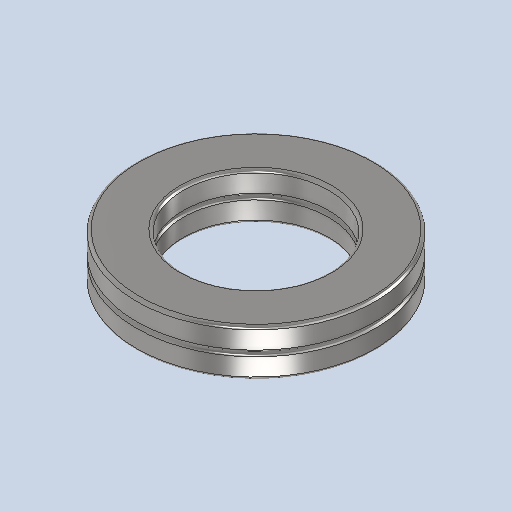
# Autodesk Inventor part: RB2508UUC0
Saved by Autodesk Inventor 2024.2 (Build 282272000, 272)
## iProperties
Created: 2024-01-04
Part Number: RB2508UUC0
Material: Generic
Document SubType Name: Modeling
Designer: Masato Kubotera
Density: 7.58662 g/cm^3
Appearance: Semi-Polished
Mass: 50 g
Surface Area: 33.4688 cm^2
Volume: 6.59055 cm^3
Catalog Web Link: https://jp.misumi-ec.com/vona2/detail/221000091353/?ProductCode=RB2508UUC0
Vendor: THK
Author: Masato Kubotera
Autodesk Inventor part; units mm, degrees
ref_plane "YZ Plane" through (0, 0, 0) normal (1, 0, 0) x (0, 1, 0)
ref_plane "XZ Plane" through (0, 0, 0) normal (0, 1, 0) x (-1, 0, 0)
ref_plane "XY Plane" through (0, 0, 0) normal (0, 0, 1) x (1, 0, 0)
sketch "Sketch1" plane through (0, 0, 0) normal (0, 1, 0) x (-1, 0, 0)
  line L0 (0, 4) -> (0, -4)
  line L1 (-13, 0) -> (-20, 0)
  line L2 (-20.5, -0.5) -> (-20.5, -3.5)
  line L3 (-20, -4) -> (-13, -4)
  line L4 (-12.5, -3.5) -> (-12.5, -0.5)
  arc A0 (-20.5, -3.5) -> (-20, -4) centre (-20, -3.5) ccw
  arc A1 (-13, -4) -> (-12.5, -3.5) centre (-13, -3.5) ccw
  arc A2 (-12.5, -0.5) -> (-13, 0) centre (-13, -0.5) ccw
  arc A3 (-20, 0) -> (-20.5, -0.5) centre (-20, -0.5) ccw
  line L5 (-20.5, 0.5) -> (-20.5, 3.5)
  line L6 (-20, 4) -> (-13, 4)
  line L7 (-12.5, 3.5) -> (-12.5, 0.5)
  arc A4 (-20, 4) -> (-20.5, 3.5) centre (-20, 3.5) ccw
  arc A5 (-12.5, 3.5) -> (-13, 4) centre (-13, 3.5) ccw
  arc A6 (-13, 0) -> (-12.5, 0.5) centre (-13, 0.5) ccw
  arc A7 (-20.5, 0.5) -> (-20, 0) centre (-20, 0.5) ccw
  point P0 (0, 0)
  dimension "d0" = 0.5
  dimension "d1" = 25
  dimension "d2" = 41
  dimension "d4" = 8
  constraints: 16 end point, 16 point on circle, 10 symmetric about line, 8 centre point, 8 tangent, 3 equal radius, 3 point on line, 2 parallel, 1 horizontal, 1 midpoint, 1 perpendicular, 1 vertical, 4 other
  measures "d0" radius of A0
  measures "d1" diameter of L4 L0
  measures "d2" diameter of L2 L0
  measures "d4" distance between parallel lines of L3 L6
revolve "Revolution1" add sketch "Sketch1" angle 360 about axis through (0, 0, 4) along (0, 0, -1)
body "Solid1"
